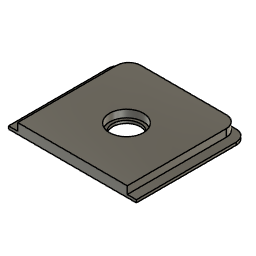
Camison (Autodesk Fusion 360 archive; units mm, degrees)
design "tapa trasera"
Autodesk Fusion 360 part; units mm, degrees
sketch "Boceto2" plane through (0, 0, 0) normal (0, 0, 1) x (1, 0, 0)
  circle A0 centre (0, 0) radius 11.25
  circle A1 centre (0, 0) radius 9.25
  line L0 (-42.6, 38) -> (42.6, 38)
  line L1 (42.6, 38) -> (42.6, -39)
  line L2 (42.6, -39) -> (-42.6, -39)
  line L3 (-42.6, -39) -> (-42.6, 38)
  line L4 (-36.5, 38) -> (-36.5, -39)
  line L5 (36.5, 38) -> (36.5, -39)
  line L6 (36.5, -0.5) -> (42.6, -0.5)
  line L7 (-36.5, -0.5) -> (-42.6, -0.5)
  circle A2 centre (35.1, 30.5) radius 7.5
  circle A3 centre (-35.1, 30.5) radius 7.5
  line L8 (42.6, -36) -> (-42.6, -36)
  dimension "d1" = 22.5
  dimension "d3" = 2
  dimension "d4" = 39
  dimension "d5" = 77
  dimension "d6" = 85.2
  dimension "d7" = 42.6
  dimension "d14" = 73
  dimension "d15" = 15
  dimension "d16" = 3
  constraint coincident A0.centre A1.centre
  constraint horizontal L0
  constraint vertical L1
  constraint horizontal L2
  constraint vertical L3
  constraint coincident L0 L4.start
  constraint coincident L2 L4.end
  constraint perpendicular L2 L4
  constraint coincident L0 L5.start
  constraint coincident L2 L5.end
  constraint perpendicular L2 L5
  constraint midpoint L5 L6.start
  constraint midpoint L1 L6.end
  constraint midpoint L4 L7.start
  constraint midpoint L3 L7.end
  constraint equal L6 L7
  constraint tangent L0 A2
  constraint tangent L3 A3
  constraint tangent L0 A3
  constraint tangent L1 A2
  constraint horizontal A2.centre A3.centre
  constraint coincident L1 L8.start
  constraint coincident L3 L8.end
  constraint horizontal L8
  measures "d1" diameter of A0
  measures "d3" distance of A0 A1
  measures "d4" distance of A0.centre L2
  measures "d5" distance of L0.start L2.end
  measures "d6" distance of L0.start L0.end
  measures "d7" distance of A0.centre L3
  measures "d14" distance of L4 L5
  measures "d15" diameter of A2
  measures "d16" distance of L2 L8
extrude "Extruir1" add sketch "Boceto2" along normal blind 5 contours L0 L4 A3 | L0 L4 L5 A2 A3 L8 | L4 A3 | L0 L5 A2 | L5 A2 picked at (-31.7419, 29.782) picked at (33.9293, 28.3684)
extrude "Extruir2" add sketch "Boceto2" against normal blind 1.8 contours A0 | L3 L4 L7 A3 | L4 A3 | L0 L4 L5 A2 A3 L8 | L4 A3 | L3 L4 L7 L8 | L5 A2 | L5 A2 | L1 L5 L6 A2 | L1 L5 L6 L8
fillet "Empalme1" radius 8 2 edges at (36.5, 38, 2.5) (-36.5, 38, 2.5)
fillet "Empalme2" [rolled back] radius 10
equation "d7 = d6 / 2"
equation "d14 = 74 mm - 1 mm"

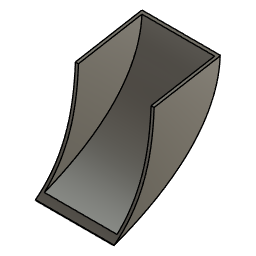
design "tobogan"
Autodesk Fusion 360 part; units mm, degrees
sketch "Boceto1" plane through (0, 0, 0) normal (1, 0, 0) x (0, 1, 0)
  line L0 (0, 0) -> (0, 40)
  spline S0 degree 5 poles (0, 0) (0, -5.3819) (-1.1773, -15.7689) (-6.475, -30.2193) (-20.0472, -47.2186) (-44.7749, -64.6171) (-73.3576, -78.0806) (-101.7766, -87.5841) (-126.6232, -93.3139) (-145.7025, -95.8198) (-159.0947, -96.3721) (-167.2377, -96.8348) (-173.1429, -97.9971) (-177.1944, -99.2523) (-179.2486, -100) knots 0 0 0 0 0 0 0.1 0.2 0.3 0.4 0.5 0.6 0.7 0.8 0.9 1 1 1 1 1 1
  line L1 (-179.2486, -100) -> (-258.9631, -129.0137) construction
  line L2 (-258.9631, -129.0137) -> (-18.0072, -129.0137) construction
  point P0 (-138.6504, -94.6835)
  dimension "d20" = 40
  dimension "d21" = 100
  dimension "d48" = 20
  constraint coincident L0.start S0.start
  constraint vertical L0
  constraint horizontal L2
  measures "d20" distance of L0.start L0.end
  measures "d21" distance of L0.start S0.end
  measures "d48" angle of L1 L2
ref_plane "PlanoDeObra1" through (0, 0, 40) normal (0, 0, 1) x (1, 0, 0)
sketch "Boceto3" plane through (0, 0, 40) normal (0, 0, 1) x (1, 0, 0)
  line L0 (36, 32.5) -> (-36, 32.5)
  line L1 (-36, 32.5) -> (-36, -32.5)
  line L2 (-36, -32.5) -> (36, -32.5)
  line L3 (36, -32.5) -> (36, 32.5)
  line L4 (36, 32.5) -> (-36, -32.5) construction
  line L5 (-36, 32.5) -> (36, -32.5) construction
  line L6 (-36, -32.5) -> (-38.5, -32.5)
  line L7 (-39, -32) -> (-39, 35)
  line L8 (-38.5, 35.5) -> (38.5, 35.5)
  line L9 (39, 35) -> (39, -32)
  line L10 (38.5, -32.5) -> (36, -32.5)
  line L11 (-36, 32.5) -> (-36, 35.5) construction
  arc A0 (-38.5, 35.5) -> (-39, 35) centre (-38.5, 35) ccw
  arc A1 (39, 35) -> (38.5, 35.5) centre (38.5, 35) ccw
  arc A2 (38.5, -32.5) -> (39, -32) centre (38.5, -32) ccw
  arc A3 (-39, -32) -> (-38.5, -32.5) centre (-38.5, -32) ccw
  line L12 (36, 32.5) -> (39, 32.5)
  line L13 (-36, 32.5) -> (-39, 32.5) construction
  dimension "d6" = 72
  dimension "d7" = 65
  dimension "d8" = 0.5
  dimension "d16" = 3
  constraint horizontal L0
  constraint perpendicular L0 L1
  constraint parallel L0 L2
  constraint parallel L1 L3
  constraint coincident L4 origin
  constraint coincident L5 origin
  constraint perpendicular L1 L6
  constraint perpendicular L6 L7
  constraint perpendicular L7 L8
  constraint horizontal L10
  constraint vertical L9
  constraint coincident L8 L11.end
  constraint perpendicular L8 L11
  constraint tangent L7 A0
  constraint tangent L8 A0
  constraint tangent L8 A1
  constraint tangent L9 A1
  constraint equal A0 A1
  constraint tangent L9 A2
  constraint tangent L10 A2
  constraint equal A0 A2
  constraint tangent L6 A3
  constraint tangent L7 A3
  constraint equal A0 A3
  constraint coincident L9 L12.end
  constraint perpendicular L9 L12
  constraint coincident L7 L13.end
  constraint perpendicular L7 L13
  constraint equal L12 L13
  constraint equal L11 L13
  measures "d6" distance of L0.start L0.end
  measures "d7" distance of L0.start L2.end
  measures "d8" radius of A0
  measures "d16" distance of L0.start L12.end
sweep "Barrido2" add profiles "Boceto3" path "Boceto1" along S0 L0 section 1 contours L3 L9 L10 A2 L12 | L0 L1 L6 L7 L8 L9 A0 A1 A3 L12
sketch "Boceto6" plane through (0, 0, 0) normal (1, 0, 0) x (0, 1, 0)
sketch "Boceto7" plane through (0, 0, 0) normal (1, 0, 0) x (0, 1, 0)
  line L0 (-907.6871, 257.2787) -> (-70, 257.2787)
  line L1 (-70, 257.2787) -> (-70, -499.7568)
  line L2 (-70, -499.7568) -> (-907.6871, -499.7568)
  line L3 (-907.6871, -499.7568) -> (-907.6871, 257.2787)
  dimension "d41" = 70
  constraint horizontal L0
  constraint vertical L1
  constraint horizontal L2
  constraint vertical L3
  measures "d41" distance of origin L1
extrude "Extruir3" cut sketch "Boceto7" along normal mid plane 160
sketch "Boceto5" plane through (0, 0, 0) normal (0, 1, 0) x (1, 0, 0)
  circle A0 centre (0, -38) radius 38
  line L0 (-38, -38) -> (38, -38)
  line L1 (-38, 0) -> (38, 0)
  line L2 (-38, -38) -> (-38, 0)
  line L3 (38, -38) -> (38, 0)
  dimension "d37" = 76
  dimension "d38" = 38
  constraint vertical origin A0.centre
  constraint horizontal L0
  constraint midpoint A0.centre L0
  constraint horizontal L1
  constraint tangent A0 L1
  constraint vertical L2
  constraint vertical L3
  constraint tangent A0 L3
  measures "d37" diameter of A0
  measures "d38" distance of origin A0.centre
extrude "Extruir2" cut sketch "Boceto5" along normal mid plane 90
ref_plane "PlanoDeObra2" through (0, 0, -120) normal (0, 0, 1) x (1, 0, 0)
sketch "Boceto12" plane through (39, 0, 0) normal (1, 0, 0) x (0, 1, 0)
  line L0 (-70, -40.4408) -> (-70, -113.3302)
  spline S0 degree 3 poles (35, 0) (35, -4.6734) (34.6572, -9.358) (33.9563, -13.9779) (33.2787, -18.4444) (32.2664, -22.8485) (30.9439, -27.1206) (28.4177, -35.2814) (24.7568, -42.9303) (20.3537, -49.8469) (16.2396, -56.3097) (11.4915, -62.1501) (6.3756, -67.4384) (1.5954, -72.3796) (-3.5096, -76.8471) (-8.8098, -80.936) (-18.5951, -88.4851) (-29.0461, -94.7667) (-39.626, -100.1604) (-48.8344, -104.8548) (-58.1454, -108.8649) (-67.2443, -112.3038) (-68.1651, -112.6518) (-69.0838, -112.9939) (-70, -113.3302) knots 0 0 0 0 0.033206 0.033206 0.033206 0.065309 0.065309 0.065309 0.126634 0.126634 0.126634 0.183935 0.183935 0.183935 0.237477 0.237477 0.237477 0.336328 0.336328 0.336328 0.422364 0.422364 0.422364 0.431071 0.431071 0.431071 0.431071
  line L1 (35, 0) -> (35, 40)
  line L2 (35, 40) -> (-32, 40)
  line L3 (-32, 40) -> (-32, 0)
  spline S1 degree 3 poles (-32, 0) (-32, -1.4288) (-32.1016, -2.715) (-32.2856, -3.9276) (-32.6371, -6.2441) (-33.2708, -8.3187) (-34.3334, -10.5662) (-35.3262, -12.6662) (-36.7197, -14.9138) (-38.6609, -17.3318) (-40.4748, -19.5912) (-42.7665, -21.9859) (-45.5242, -24.42) (-48.101, -26.6943) (-51.0804, -28.9997) (-54.3836, -31.2619) (-59.0465, -34.4554) (-64.3517, -37.5587) (-70, -40.4408) knots 0 0 0 0 0.033206 0.033206 0.033206 0.096637 0.096637 0.096637 0.155907 0.155907 0.155907 0.211288 0.211288 0.211288 0.263035 0.263035 0.263035 0.336085 0.336085 0.336085 0.336085
  spline S2 degree 5 poles (-32, 40) (-31.6354, 35.5748) (-30.9974, 26.8344) (-30.3138, 14.0542) (-29.9582, -2.3146) (-30.5095, -21.5725) (-32.1652, -39.4961) (-35.0537, -55.9303) (-39.2944, -70.731) (-44.943, -83.8306) (-51.9475, -95.2922) (-58.5701, -103.2303) (-64.0781, -108.5303) (-67.9866, -111.7779) (-70, -113.3302) knots 0 0 0 0 0 0 0.1 0.2 0.3 0.4 0.5 0.6 0.7 0.8 0.9 1 1 1 1 1 1
  line L4 (-33.2437, -44.3921) -> (-90.7775, -76.7738)
  line L5 (-90.7775, -76.7738) -> (-70, -113.3302)
  line L6 (53.9678, 0) -> (-90.7775, -25.5225)
  line L7 (53.9678, 0) -> (53.9678, 107.8057)
  line L8 (53.9678, 107.8057) -> (-90.7775, 107.8057)
  line L9 (-90.7775, 107.8057) -> (-90.7775, -76.7738)
  point P0 (-38.7653, -67.7304)
  dimension "d55" = 100
  constraint coincident L2.end L3.start
  constraint coincident L0.end S0.end
  constraint coincident S2 L4.start
  constraint vertical L9
  constraint vertical L7
  constraint horizontal L8
  constraint coincident L6.end L9
  constraint horizontal origin L6.start
  measures "d55" angle of L6 L7
extrude "Extruir5" cut sketch "Boceto12" against normal blind 140 contours L0 S1 S2 L4 L6 | L0 S1 L4 L6 L9 | L0 S2 L4 | L0 L4 L5 | S0 L1 L2 L3 S1 L6 L7 L8 L9 | L3 S1 S2 L6 | S0 L1 L2 S2 L6
sketch "Boceto11" plane through (0, 0, 0) normal (0, 0, 1) x (1, 0, 0)
  circle A0 centre (-17.2307, -70.0803) radius 52
  point P0 (17.5, -31.3791)
  point P1 (-38.5, -22.6291)
  dimension "d51" = 104
  constraint coincident A0 P0
  constraint coincident A0 P1
  measures "d51" diameter of A0

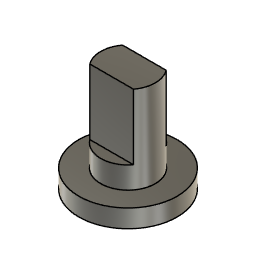
design "Eje motor"
Autodesk Fusion 360 part; units mm, degrees
sketch "Boceto1" plane through (0, 0, 0) normal (0, 0, 1) x (1, 0, 0)
  circle A0 centre (0, 0) radius 2.5
  line L0 (-2, 1.5) -> (2, 1.5)
  circle A1 centre (0, 0) radius 4.5
  line L1 (-2, -1.5) -> (2, -1.5)
  dimension "d1" = 5
  dimension "d2" = 1.5
  dimension "d3" = 9
  dimension "d10" = 3
  constraint coincident A0.centre A1.centre
  constraint coincident A0 L0.start
  constraint coincident A0 L0.end
  constraint horizontal L0
  constraint concentric A0 A1
  constraint coincident A0 L1.start
  constraint coincident A0 L1.end
  constraint horizontal L1
  measures "d1" diameter of A0
  measures "d2" distance of A0.centre L0
  measures "d3" diameter of A1
  measures "d10" distance of L0 L1
extrude "Extruir1" add sketch "Boceto1" along normal blind 8 contours A0 L0 L1 makes body 1
extrude "Extruir2" add sketch "Boceto1" along normal blind 2 contours A0 L0 | A0 L1 bodies 1
extrude "Extruir3" add sketch "Boceto1" against normal blind 1.65 separate body makes body 2
equation "d2 = d10 / 2"

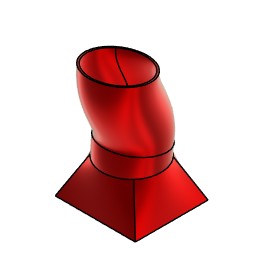
design "Tolva de alimentacion"
Autodesk Fusion 360 part; units mm, degrees
sketch "Boceto1" plane through (0, 0, 0) normal (0, 0, 1) x (1, 0, 0)
  circle A0 centre (0, 0) radius 30
  circle A1 centre (0, 0) radius 32
  dimension "d12" = 2
  dimension "d13" = 60
  constraint coincident A0.centre A1.centre
  measures "d12" distance of A0 A1
  measures "d13" diameter of A0
ref_plane "PlanoDeObra1" through (0, 0, -40) normal (0, 0, 1) x (1, 0, 0)
sketch "Boceto2" plane through (0, 0, -40) normal (0, 0, 1) x (1, 0, 0)
  line L0 (-40, 36) -> (-40, -36)
  line L1 (40, 36) -> (40, -36)
  line L2 (-40, 36) -> (40, 36)
  line L3 (-40, -36) -> (40, -36)
  line L4 (43.5, 39.5) -> (43.5, -39.5)
  line L5 (-43.5, -39.5) -> (43.5, -39.5)
  line L6 (-43.5, 39.5) -> (-43.5, -39.5)
  line L7 (-43.5, 39.5) -> (43.5, 39.5)
  line L8 (0, 36) -> (0, -36) construction
  dimension "d2" = 3.5
  dimension "d4" = 72
  dimension "d5" = 87
  constraint vertical L1
  constraint horizontal L2
  constraint horizontal L3
  constraint vertical L0
  constraint midpoint L2 L8.start
  constraint midpoint L3 L8.end
  constraint midpoint L8 origin
  measures "d4" distance of L1.start L1.end
  measures "d5" distance of L4.start L6.start
loft "Solevación1" add profiles "Boceto2", "Boceto1" section 1 section 2
loft "Solevación2" cut profiles "Boceto2", "Boceto1" section 1 contours L0 L1 L2 L3 section 2 contours A0
sketch "Boceto5" plane through (0, 0, 0) normal (1, 0, 0) x (0, 1, 0)
  arc A0 (1.4235, 16.2702) -> (0, 0) centre (93.6965, 0) ccw
  dimension "d22" = 10
  constraint coincident A0.end origin
  constraint horizontal A0.end A0.centre
  measures "d22" angle of A0.end A0.start A0.centre
sweep "Barrido1" add 1 faces at (24.1943, 19.793, 0) path "Boceto5" along A0
sketch "Boceto6" plane through (0, 0, 0) normal (1, 0, 0) x (0, 1, 0)
  arc A0 (1.4235, 16.2702) -> (0, 0) centre (93.6965, 0) ccw
  line L0 (-14.758, 90.6645) -> (-25.6524, 20.4726) construction
  line L1 (-25.6524, 20.4726) -> (1.4235, 16.2702) construction
  spline S0 degree 5 poles (-14.758, 90.6645) (-15.0151, 89.0086) (-15.3594, 85.682) (-15.3667, 80.6478) (-14.4239, 73.8789) (-12.0247, 65.4963) (-8.8804, 57.4) (-5.4982, 49.7683) (-2.3587, 42.6952) (0.1604, 36.091) (1.7957, 29.6992) (2.2467, 24.5147) (2.049, 20.4682) (1.6727, 17.684) (1.4235, 16.2702) knots 0 0 0 0 0 0 0.1 0.2 0.3 0.4 0.5 0.6 0.7 0.8 0.9 1 1 1 1 1 1
  line L2 (3.1484, 26.0527) -> (-0.3015, 6.4877)
  point P0 (1.4235, 16.2702)
  point P1 (-4.056, 46.4663)
  dimension "d23" = 27.4
  constraint coincident P0 A0.start
  constraint perpendicular L0 L1
  constraint midpoint P0 L2
  constraint tangent A0 L2
  measures "d23" distance of L0.end P0
sweep "Barrido2" add 1 faces at (4.2954, -29.0665, 21.6464) path "Boceto6" along S0
sketch "Boceto4" plane through (0, 0, 0) normal (1, 0, 0) x (0, 1, 0)
  circle A0 centre (0, -70) radius 20.5
  line L0 (23, -70) -> (-23, -70)
  dimension "d3" = 41
  constraint vertical A0.centre origin
  constraint coincident A0.centre L0
  measures "d3" diameter of A0
extrude "Extruir1" [suppressed]
equation "d4 = 79 mm - 2 * d2"
equation "d5 = 80 mm + 2 * d2"

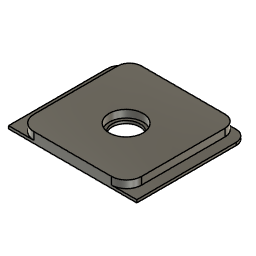
design "tapa1"
Autodesk Fusion 360 part; units mm, degrees
sketch "Boceto2" plane through (0, 0, 0) normal (0, 0, 1) x (1, 0, 0)
  circle A0 centre (0, 0) radius 11.25
  circle A1 centre (0, 0) radius 9.25
  line L0 (-42.6, 38) -> (42.6, 38)
  line L1 (42.6, 38) -> (42.6, -39)
  line L2 (42.6, -39) -> (-42.6, -39)
  line L3 (-42.6, -39) -> (-42.6, 38)
  line L4 (-35.75, 38) -> (-35.75, -39)
  line L5 (35.75, 38) -> (35.75, -39)
  line L6 (35.75, -0.5) -> (42.6, -0.5)
  line L7 (-35.75, -0.5) -> (-42.6, -0.5)
  circle A2 centre (35.1, 30.5) radius 7.5
  circle A3 centre (-35.1, 30.5) radius 7.5
  line L8 (42.6, -35.5) -> (-42.6, -35.5)
  dimension "d1" = 22.5
  dimension "d3" = 2
  dimension "d4" = 39
  dimension "d5" = 77
  dimension "d6" = 85.2
  dimension "d7" = 42.6
  dimension "d14" = 71.5
  dimension "d15" = 15
  dimension "d16" = 3.5
  constraint coincident A0.centre A1.centre
  constraint horizontal L0
  constraint vertical L1
  constraint horizontal L2
  constraint vertical L3
  constraint coincident L0 L4.start
  constraint coincident L2 L4.end
  constraint perpendicular L2 L4
  constraint coincident L0 L5.start
  constraint coincident L2 L5.end
  constraint perpendicular L2 L5
  constraint midpoint L5 L6.start
  constraint midpoint L1 L6.end
  constraint midpoint L4 L7.start
  constraint midpoint L3 L7.end
  constraint equal L6 L7
  constraint tangent L0 A2
  constraint tangent L3 A3
  constraint tangent L0 A3
  constraint tangent L1 A2
  constraint horizontal A2.centre A3.centre
  constraint coincident L1 L8.start
  constraint coincident L3 L8.end
  constraint horizontal L8
  measures "d1" diameter of A0
  measures "d3" distance of A0 A1
  measures "d4" distance of A0.centre L2
  measures "d5" distance of L0.start L2.end
  measures "d6" distance of L0.start L0.end
  measures "d7" distance of A0.centre L3
  measures "d14" distance of L4 L5
  measures "d15" diameter of A2
  measures "d16" distance of L2 L8
extrude "Extruir1" add sketch "Boceto2" along normal blind 5 contours L0 L4 A3 | L0 L4 L5 A2 A3 L8 | L4 A3 | L0 L5 A2 | L5 A2 picked at (-32.8167, 30.5094) picked at (33.1671, 32.0923)
extrude "Extruir2" add sketch "Boceto2" against normal blind 1.8 contours A0 | L3 L4 L7 A3 | L4 A3 | L0 L4 L5 A2 A3 L8 | L4 A3 | L3 L4 L7 L8 | L5 A2 | L5 A2 | L1 L5 L6 A2 | L1 L5 L6 L8
fillet "Empalme1" radius 8 2 edges at (35.75, 38, 2.5) (-35.75, 38, 2.5)
fillet "Empalme2" radius 10 2 edges at (-35.75, -35.5, 2.5) (35.75, -35.5, 2.5)
equation "d7 = d6 / 2"
